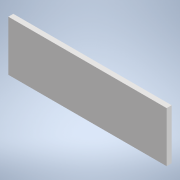
# Autodesk Inventor part: LinePCB
Saved by Autodesk Inventor 2021 (Build 250183000, 183)
## iProperties
Created: 2021-02-19
Part Number: LinePCB
Material: FR4
Document SubType Name: Modeling
Designer: James
Density: 1 g/cm^3
Appearance: Default
Author: James
Autodesk Inventor part; units mm, degrees
ref_plane "YZ Plane" through (0, 0, 0) normal (1, 0, 0) x (0, 1, 0)
ref_plane "XZ Plane" through (0, 0, 0) normal (0, 1, 0) x (-1, 0, 0)
ref_plane "XY Plane" through (0, 0, 0) normal (0, 0, 1) x (1, 0, 0)
sketch "Sketch1" plane through (0, 0, 0) normal (0, 0, 1) x (1, 0, 0)
  arc A0 (-35.3193, 63.4215) -> (-33.3193, 61.4215) centre (-33.3193, 63.4215) ccw projected
  circle A1 centre (15.1807, 64.4604) radius 1.75 projected
  circle A2 centre (15.1807, 134.4604) radius 1.75 projected
  circle A3 centre (-24.8193, 64.4604) radius 1.75 projected
  circle A4 centre (-24.8193, 134.4604) radius 1.75 projected
  circle A5 centre (18.1807, 121.7104) radius 2.5 projected
  circle A6 centre (-27.8193, 77.2104) radius 2.5 projected
  circle A7 centre (-4.8193, 139.4604) radius 2.5 projected
  circle A8 centre (18.1807, 77.2104) radius 2.5 projected
  circle A9 centre (-4.8193, 59.4604) radius 2.5 projected
  circle A10 centre (-27.8193, 121.7104) radius 2.5 projected
  arc A11 (-35.3193, 63.4215) -> (-33.3193, 61.4215) centre (-33.3193, 63.4215) ccw projected
  line L0 (-32.8356, 61.4215) -> (-33.3193, 61.4215) projected
  arc A12 (-26.8356, 55.4215) -> (-32.8356, 61.4215) centre (-32.8356, 55.4215) ccw projected
  line L1 (-26.8356, 54.9604) -> (-26.8356, 55.4215)
  arc A13 (-26.8356, 54.9604) -> (-24.8356, 52.9604) centre (-24.8356, 54.9604) ccw projected
  line L2 (15.2262, 52.9604) -> (-24.8356, 52.9604) projected
  arc A14 (15.2262, 52.9604) -> (17.2262, 54.9604) centre (15.2262, 54.9604) ccw projected
  line L3 (17.2262, 55.4604) -> (17.2262, 54.9604) projected
  arc A15 (23.2262, 61.4604) -> (17.2262, 55.4604) centre (23.2262, 55.4604) ccw projected
  line L4 (23.6807, 61.4604) -> (23.2262, 61.4604) projected
  arc A16 (23.6807, 61.4604) -> (25.6807, 63.4604) centre (23.6807, 63.4604) ccw projected
  line L5 (25.6807, 135.4604) -> (25.6807, 63.4604) projected
  arc A17 (25.6807, 135.4604) -> (23.6807, 137.4604) centre (23.6807, 135.4604) ccw projected
  line L6 (23.1807, 137.4604) -> (23.6807, 137.4604) projected
  arc A18 (17.1807, 143.4604) -> (23.1807, 137.4604) centre (23.1807, 143.4604) ccw projected
  line L7 (17.1807, 143.9604) -> (17.1807, 143.4604) projected
  arc A19 (17.1807, 143.9604) -> (15.1807, 145.9604) centre (15.1807, 143.9604) ccw projected
  line L8 (-24.8193, 145.9604) -> (15.1807, 145.9604) projected
  arc A20 (-24.8193, 145.9604) -> (-26.8193, 143.9604) centre (-24.8193, 143.9604) ccw projected
  line L9 (-26.8193, 143.4604) -> (-26.8193, 143.9604) projected
  arc A21 (-32.8193, 137.4604) -> (-26.8193, 143.4604) centre (-32.8193, 143.4604) ccw projected
  line L10 (-33.3193, 137.4604) -> (-32.8193, 137.4604) projected
  arc A22 (-33.3193, 137.4604) -> (-35.3193, 135.4604) centre (-33.3193, 135.4604) ccw projected
  line L11 (-35.3193, 63.4215) -> (-35.3193, 135.4604) projected
  circle A23 centre (23.1807, 55.4604) radius 2 projected
  circle A24 centre (-32.8193, 55.4604) radius 2 projected
  line L12 (-34.8193, 69.4604) -> (25.1807, 69.4604) projected
  circle A25 centre (-24.8193, 64.4604) radius 1.75 projected
  circle A26 centre (15.1807, 64.4604) radius 1.75 projected
  line L13 (-24.8193, 66.2104) -> (15.1807, 66.2104)
  line L14 (15.1807, 66.2104) -> (15.1807, 53.5104)
  line L15 (15.1807, 53.5104) -> (-24.8193, 53.5104)
  line L16 (-24.8193, 53.5104) -> (-24.8193, 66.2104)
  point P0 (0, 0)
  dimension "d4" = 12.7
  constraints: 10 end point, 2 parallel, 2 vertical alignment, 1 horizontal, 1 perpendicular, 1 point on line, 1 tangent, 2 other
  measures "d4" distance of L13.end L14.end
extrude "Extrusion1" add sketch "Sketch1" along normal blind 1.6 contours L14 A1 | A1 L14 L15 L16 A3 L13 | A3 L16 | A9 picked at (14.5228, 63.957) picked at (-24.196, 64.9165)
body "Solid1"
